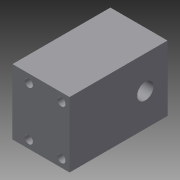
# Autodesk Inventor part: Linear Bearing
Saved by Autodesk Inventor 2014 (Build 180170000, 170)
## iProperties
Created: 2014-02-25
Part Number: Linear Bearing
Material: Generic
Document SubType Name: Modeling
Designer: Nitesh
Density: 1 g/cm^3
Appearance: Default
Author: Nitesh
Autodesk Inventor part; units mm, degrees
ref_plane "YZ Plane" through (0, 0, 0) normal (1, 0, 0) x (0, 1, 0)
ref_plane "XZ Plane" through (0, 0, 0) normal (0, 1, 0) x (-1, 0, 0)
ref_plane "XY Plane" through (0, 0, 0) normal (0, 0, 1) x (1, 0, 0)
sketch "Sketch1" plane through (0, 0, 0) normal (1, 0, 0) x (0, 1, 0)
  line L0 (0, 0) -> (50.8, 0)
  line L1 (50.8, 0) -> (50.8, 76.2)
  line L2 (50.8, 76.2) -> (0, 76.2)
  line L3 (0, 76.2) -> (0, 0)
  dimension "d0" = 76.2
  dimension "d1" = 50.8
  constraints: 8 end point, 2 parallel, 1 horizontal, 1 perpendicular
  measures "d0" distance of L2.end L0.start
  measures "d1" distance of L1.end L2.end
extrude "Extrusion1" add sketch "Sketch1" along normal blind 44.45
sketch "Sketch2" plane through (44.45, 0, 0) normal (1, 0, 0) x (0, 0, -1)
  line L0 (0, 50.8) -> (-76.2, 50.8) projected
  line L1 (-76.2, 50.8) -> (-76.2, 0) projected
  circle A0 centre (-17.272, 25.4) radius 6.35
  dimension "d4" = 12.7
  dimension "d5" = 25.4
  dimension "d6" = 58.928
  constraints: 1 centre point
  measures "d4" diameter of A0
  measures "d5" distance from line of L0 A0.centre
  measures "d6" distance from line of L1 A0.centre
extrude "Extrusion2" cut sketch "Sketch2" against normal blind 38.1
sketch "Sketch3" plane through (0, 0, 0) normal (0, 0, -1) x (-1, 0, 0)
  line L0 (0, 0) -> (0, 50.8) projected
  line L1 (0, 50.8) -> (-44.45, 50.8) projected
  line L2 (-44.45, 0) -> (-44.45, 50.8) projected
  line L3 (0, 0) -> (-44.45, 0) projected
  point P0 (-38.1, 44.45)
  point P1 (-12.7, 44.45)
  point P2 (-12.7, 6.35)
  point P3 (-38.1, 6.35)
  dimension "d9" = 6.35
  dimension "d10" = 6.35
  dimension "d11" = 6.35
  dimension "d12" = 12.7
  dimension "d13" = 12.7
  dimension "d14" = 6.35
  dimension "d15" = 6.35
  dimension "d16" = 6.35
  measures "d9" distance from line of L2 point (-38.1, 44.45)
  measures "d10" distance from line of L1 point (-38.1, 44.45)
  measures "d11" distance from line of L1 point (-12.7, 44.45)
  measures "d12" distance from line of L0 point (-12.7, 44.45)
  measures "d13" distance from line of L0 point (-12.7, 6.35)
  measures "d14" distance from line of L3 point (-12.7, 6.35)
  measures "d15" distance from line of L2 point (-38.1, 6.35)
  measures "d16" distance from line of L3 point (-38.1, 6.35)
hole "Hole1" at (38.1, 44.45, 0) at (12.7, 44.45, 0) at (12.7, 6.35, 0) at (38.1, 6.35, 0) direction (0, 0, 1) diameter 6.35 end through all
body "Solid1"
